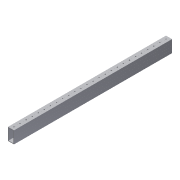
# Autodesk Inventor part: VersaFrame practice end rail 26 in
Saved by Autodesk Inventor 2015 (Build 190159000, 159)
## iProperties
Created: 2013-12-18
Part Number: VersaFrame practice end rail 26 in
Material: Aluminum 6061
Document SubType Name: Modeling
Designer: Niemitalo_Dan
Density: 1 g/cm^3
Appearance: Aluminum - Flat
Author: Niemitalo_Dan
Autodesk Inventor part; units mm, degrees
ref_plane "YZ Plane" through (0, 0, 0) normal (1, 0, 0) x (0, 1, 0)
ref_plane "XZ Plane" through (0, 0, 0) normal (0, 1, 0) x (-1, 0, 0)
ref_plane "XY Plane" through (0, 0, 0) normal (0, 0, 1) x (1, 0, 0)
sketch "VersaFrameProfile" plane through (0, 0, 0) normal (0, 0, 1) x (1, 0, 0)
  line L0 (12.7, 0.0762) -> (12.7, 12.6238)
  line L1 (-12.7, 12.6238) -> (-12.7, 0.0762)
  line L2 (-12.7, 0.0762) -> (-12.6238, 0)
  line L3 (12.6238, 0) -> (12.7, 0.0762)
  line L4 (-12.6238, 0) -> (-12.7, -0.0762)
  line L5 (12.7, -0.0762) -> (12.6238, 0)
  line L6 (10.16, 22.86) -> (10.16, -22.86)
  line L7 (-10.16, -22.86) -> (-10.16, 22.86)
  line L8 (12.7, -12.6238) -> (12.7, -0.0762)
  line L9 (-12.7, -0.0762) -> (-12.7, -12.6238)
  line L10 (-12.7, 12.7762) -> (-12.6238, 12.7)
  line L11 (12.7, 12.6238) -> (12.6238, 12.7)
  line L12 (12.6238, 12.7) -> (12.7, 12.7762)
  line L13 (-12.7, 25.4) -> (-12.7, 12.7762)
  line L14 (0, 25.3238) -> (-0.0762, 25.4)
  line L15 (0.0762, 25.4) -> (0, 25.3238)
  line L16 (-10.16, 22.86) -> (10.16, 22.86)
  line L17 (12.7, 12.7762) -> (12.7, 25.4)
  line L18 (12.7, 25.4) -> (0.0762, 25.4)
  line L19 (-0.0762, 25.4) -> (-12.7, 25.4)
  line L20 (-12.6238, 12.7) -> (-12.7, 12.6238)
  line L21 (12.6238, -12.7) -> (12.7, -12.6238)
  line L22 (-12.7, -12.6238) -> (-12.6238, -12.7)
  line L23 (-12.6238, -12.7) -> (-12.7, -12.7762)
  line L24 (12.7, -12.7762) -> (12.6238, -12.7)
  line L25 (-12.7, -12.7762) -> (-12.7, -25.4)
  line L26 (-12.7, -25.4) -> (-0.0762, -25.4)
  line L27 (10.16, -22.86) -> (-10.16, -22.86)
  line L28 (-0.0762, -25.4) -> (0, -25.3238)
  line L29 (12.7, -25.4) -> (12.7, -12.7762)
  line L30 (0.0762, -25.4) -> (12.7, -25.4)
  line L31 (0, -25.3238) -> (0.0762, -25.4)
  point P0 (0, 0)
  point P1 (0, 0)
sketch "Sketch1" plane through (0, 0, 0) normal (0, 0, 1) x (1, 0, 0)
  line L0 (12.7, 0.0762) -> (12.7, 12.6238)
  line L1 (-12.7, 12.6238) -> (-12.7, 0.0762)
  line L2 (-12.7, 0.0762) -> (-12.6238, 0)
  line L3 (12.6238, 0) -> (12.7, 0.0762)
  line L4 (-12.6238, 0) -> (-12.7, -0.0762)
  line L5 (12.7, -0.0762) -> (12.6238, 0)
  line L6 (10.16, 22.86) -> (10.16, -22.86)
  line L7 (-10.16, -22.86) -> (-10.16, 22.86)
  line L8 (12.7, -12.6238) -> (12.7, -0.0762)
  line L9 (-12.7, -0.0762) -> (-12.7, -12.6238)
  line L10 (-12.7, 12.7762) -> (-12.6238, 12.7)
  line L11 (12.7, 12.6238) -> (12.6238, 12.7)
  line L12 (12.6238, 12.7) -> (12.7, 12.7762)
  line L13 (-12.7, 25.4) -> (-12.7, 12.7762)
  line L14 (0, 25.3238) -> (-0.0762, 25.4)
  line L15 (0.0762, 25.4) -> (0, 25.3238)
  line L16 (-10.16, 22.86) -> (10.16, 22.86)
  line L17 (12.7, 12.7762) -> (12.7, 25.4)
  line L18 (12.7, 25.4) -> (0.0762, 25.4)
  line L19 (-0.0762, 25.4) -> (-12.7, 25.4)
  line L20 (-12.6238, 12.7) -> (-12.7, 12.6238)
  line L21 (12.6238, -12.7) -> (12.7, -12.6238)
  line L22 (-12.7, -12.6238) -> (-12.6238, -12.7)
  line L23 (-12.6238, -12.7) -> (-12.7, -12.7762)
  line L24 (12.7, -12.7762) -> (12.6238, -12.7)
  line L25 (-12.7, -12.7762) -> (-12.7, -25.4)
  line L26 (-12.7, -25.4) -> (-0.0762, -25.4)
  line L27 (10.16, -22.86) -> (-10.16, -22.86)
  line L28 (-0.0762, -25.4) -> (0, -25.3238)
  line L29 (12.7, -25.4) -> (12.7, -12.7762)
  line L30 (0.0762, -25.4) -> (12.7, -25.4)
  line L31 (0, -25.3238) -> (0.0762, -25.4)
  point P0 (0, 0)
  constraints: 1 other
extrude "Extrusion1" add sketch "Sketch1" along normal mid plane 1524
sketch "Sketch2" plane through (0, 0, 0) normal (0, 1, 0) x (-1, 0, 0)
  line L0 (0, 0) -> (0, 1.27) construction
  circle A0 centre (0, 12.7) radius 2.0828
  circle A1 centre (0, -12.7) radius 2.0828
  dimension "d11" = 1.27
  dimension "d12" = 4.1656
  dimension "d13" = 4.1656
  dimension "d15" = 25.4
  constraints: 3 vertical alignment, 2 centre point, 2 end point, 1 vertical
  measures "d11" distance of L0.start L0.end
  measures "d12" diameter of A0
  measures "d13" diameter of A1
  measures "d15" distance of A1.centre A0.centre
extrude "Extrusion2" cut sketch "Sketch2" along normal through all both and the other way through all
pattern_linear "Rectangular Pattern1" count 30 spacing 50.8 along (0, 0, 1) of "Extrusion2" first direction both ways yes
sketch "Sketch3" plane through (0, 0, 0) normal (0, 0, 1) x (1, 0, 0)
  line L0 (-12.7, 25.4) -> (12.7, 25.4)
  line L1 (12.7, 25.4) -> (12.7, -25.4)
  line L2 (12.7, -25.4) -> (-12.7, -25.4)
  line L3 (-12.7, -25.4) -> (-12.7, 25.4)
  point P0 (0, 0)
  point P1 (-12.7, 0)
  point P2 (0, 25.4)
  dimension "d21" = 25.4
  dimension "d22" = 50.8
  constraints: 8 end point, 2 midpoint, 2 parallel, 1 horizontal, 1 horizontal alignment, 1 perpendicular, 1 vertical alignment
  measures "d21" distance of L1.end L2.end
  measures "d22" distance of L0.end L1.end
extrude "Extrusion3" cut sketch "Sketch3" along normal mid plane 660.4 keep common part
body "Solid1"
